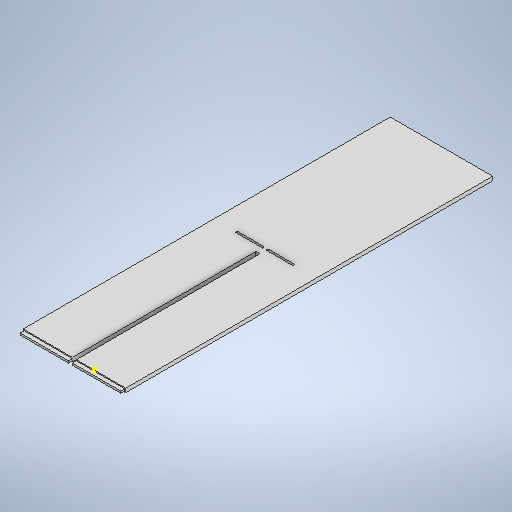
# Autodesk Inventor part: Sustainable Chair_V2 - Leg(A)_1_CPY
Saved by Autodesk Inventor 2025.2 (Build 292293000, 293)
## iProperties
Created: 2025-02-09
Part Number: Sustainable Chair_V2 - Leg(A)_1_CPY
Material: Foam Board - V3
Document SubType Name: Modeling
Designer: Dylan
Mass: 39.6007 g
Surface Area: 1188.97 cm^2
Volume: 262.027 cm^3
Density: 0.151132 g/cm^3
Appearance: Default(1)
Author: VRK99-0110
Title: Sustainable Chair_V2 - Leg(A)_1_CPY
Subject: Sustainable Chair Project
Autodesk Inventor part; units mm, degrees
ref_plane "YZ Plane" through (0, 0, 0) normal (1, 0, 0) x (0, 1, 0)
ref_plane "XZ Plane" through (0, 0, 0) normal (0, 1, 0) x (-1, 0, 0)
ref_plane "XY Plane" through (0, 0, 0) normal (0, 0, 1) x (1, 0, 0)
sketch "Sketch1" plane through (0, 0, 0) normal (0, 1, 0) x (-1, 0, 0)
  line L0 (0, 0) -> (50, 0)
  line L1 (50, 0) -> (50, -447.675)
  line L2 (50, -447.675) -> (0, -447.675)
  line L3 (0, -447.675) -> (0, 0)
  dimension "d0" = 50
  dimension "d1" = 447.675
  constraints: 8 end point, 2 parallel, 1 horizontal, 1 perpendicular
  measures "d0" distance of L1.end L2.end
  measures "d1" distance of L0.end L1.end
extrude "Extrusion1" add sketch "Sketch1" along normal blind 4.7625
sketch "Sketch2" plane through (-50, 0, 0) normal (0, 0, 1) x (1, 0, 0)
  line L0 (1.1907, 3.5648) -> (1.1907, 1.1907)
  line L1 (50, 0) -> (0, 0) projected
  line L2 (50, 4.7625) -> (0, 4.7625) projected
  line L3 (1.1907, 1.1907) -> (48.8093, 1.1907)
  line L4 (1.1907, 3.5648) -> (48.8093, 3.5648)
  line L5 (48.8093, 3.5648) -> (48.8093, 1.1907)
  line L6 (50, 0) -> (50, 4.7625) projected
  constraints: 8 end point, 1 parallel
extrude "Extrusion2" add sketch "Sketch2" along normal blind 4.7625
sketch "Sketch3" plane through (0, 4.7625, 0) normal (0, 1, 0) x (1, 0, 0)
  line L0 (-50, 447.675) -> (-50, 0) projected
  line L1 (-50, 447.675) -> (-25, 447.675)
  line L2 (0, 447.675) -> (-50, 447.675) projected
  line L3 (-25, 447.675) -> (-25, 382.675)
  line L4 (-31, 382.675) -> (-19, 382.675)
  line L5 (-31, 382.675) -> (-31, 0)
  line L6 (-1.1907, 0) -> (-48.8093, 0) projected
  line L7 (-19, 382.675) -> (-19, 0)
  line L8 (-31, 0) -> (-19, 0)
  point P0 (0, 0)
  dimension "d11" = 25
  constraints: 12 end point, 2 point on line, 2 vertical, 1 horizontal, 1 midpoint, 1 parallel, 1 perpendicular
  measures "d11" distance of L0.start L1.end
extrude "Extrusion3" cut sketch "Sketch3" against normal blind 10
sketch "Sketch4" plane through (-50, 0, 4.7625) normal (0, 0, 1) x (1, 0, 0)
  line L0 (31, 3.5648) -> (31, 1.1907) projected
  line L1 (31, 1.1907) -> (31, 3.5648)
  line L2 (19, 3.5648) -> (31, 3.5648) projected
  line L3 (31, 3.5648) -> (19, 3.5648)
  line L4 (19, 3.5648) -> (19, 1.1907)
  line L5 (19, 1.1907) -> (31, 1.1907)
  point P0 (50, 0)
  constraints: 8 end point, 3 perpendicular, 1 collinear
extrude "Extrusion4" cut sketch "Sketch4" against normal blind 10
sketch "Sketch5" plane through (0, 4.7625, 0) normal (0, 1, 0) x (1, 0, 0)
  point P0 (0, 0)
sketch "Sketch6" plane through (-31, 4.7625, -382.675) normal (0, 0, 1) x (1, 0, 0)
  line L0 (12, -4.7625) -> (0, -4.7625) projected
  line L1 (12, 0) -> (12, -4.7625) projected
  line L2 (0, 0) -> (12, 0) projected
  line L3 (0, 0) -> (0, -4.7625) projected
  point P0 (31, -4.7625)
extrude "Extrusion5" add sketch "Sketch6" along normal blind 158.838
sketch "Sketch8" plane through (-31, 4.7625, -223.837) normal (0, 0, 1) x (1, 0, 0)
  line L0 (3.6185, -4.7625) -> (3.6185, 0)
  line L1 (3.6185, 0) -> (8.3815, 0)
  line L2 (8.3815, 0) -> (8.3815, -4.7625)
  line L3 (3.6185, -4.7625) -> (8.3815, -4.7625)
  line L4 (0, -4.7625) -> (12, -4.7625) projected
  line L5 (-19, 0) -> (0, 0) projected
  line L6 (0, 0) -> (3.6185, 0)
  line L7 (12, 0) -> (0, 0) projected
  line L8 (3.6185, -4.7625) -> (0, -4.7625)
  line L9 (0, -4.7625) -> (0, 0) projected
  line L10 (0, -4.7625) -> (0, 0)
  line L11 (8.3815, 0) -> (12, 0)
  line L12 (12, -3.5718) -> (12, -4.7625) projected
  line L13 (12, -4.7625) -> (8.3815, -4.7625)
  line L14 (12, -4.7625) -> (12, 0)
  point P0 (31, -4.7625)
  dimension "d25" = 4.763
  constraints: 20 end point, 5 collinear, 3 perpendicular, 1 parallel
  measures "d25" distance of L0.end L1.end
extrude "Extrusion6" add sketch "Sketch8" along normal blind 223.837 contours L4 L9 L6 L0 | L2 L7 L14 L12 L4
sketch "Sketch9" plane through (-19, 1.1907, 0) normal (-1, 0, 0) x (0, 0, 1)
  line L0 (0, 2.374) -> (0, 0) projected
  line L1 (4.7625, 0) -> (0, 0) projected
  line L2 (4.7625, 2.374) -> (4.7625, 0) projected
  line L3 (0, 2.374) -> (4.7625, 2.374) projected
  point P0 (0, -1.1907)
extrude "Extrusion7" add sketch "Sketch9" along normal blind 15
sketch "Sketch10" plane through (-22.6185, 3.5648, 0) normal (0, 0, -1) x (-1, 0, 0)
  line L0 (4.763, -2.374) -> (4.763, 0) projected
  line L1 (0, 0) -> (4.763, 0) projected
  line L2 (0, 0) -> (0, -2.374) projected
  line L3 (0, -2.374) -> (4.763, -2.374) projected
  point P0 (-22.6185, -3.5648)
extrude "Extrusion8" cut sketch "Sketch10" against normal blind 15
sketch "Sketch14" plane through (0, 4.7625, 0) normal (0, 1, 0) x (1, 0, 0)
  line L0 (0, 447.675) -> (-50, 447.675) projected
  line L1 (0, 0) -> (0, 447.675) projected
  line L2 (-50, 447.675) -> (-50, 0) projected
  line L3 (-27.3815, 223.837) -> (-27.3815, 0) projected
  line L4 (-22.6185, 223.837) -> (-22.6185, 0) projected
  line L5 (-5, 231.488) -> (-22.6185, 231.488)
  line L6 (-22.6185, 231.488) -> (-22.6185, 233.862)
  line L7 (-22.6185, 233.862) -> (-5, 233.862)
  line L8 (-5, 231.488) -> (-5, 233.862)
  line L9 (-27.3815, 223.837) -> (-22.6185, 223.837) projected
  line L10 (-45, 231.488) -> (-27.3815, 231.488)
  line L11 (-27.3815, 231.488) -> (-27.3815, 233.862)
  line L12 (-27.3815, 233.862) -> (-45, 233.862)
  line L13 (-45, 231.488) -> (-45, 233.862)
  dimension "d35" = 2.374
  constraints: 16 end point, 1 perpendicular
  measures "d35" distance of L5.end L6.end
extrude "Extrusion9" cut sketch "Sketch14" against normal blind 10
sketch "Sketch17" plane through (0, 4.7625, 0) normal (0, 1, 0) x (1, 0, 0)
  line L0 (0, 0) -> (37.5, 0)
  line L1 (0, 447.675) -> (-50, 447.675) projected
  line L2 (0, 447.675) -> (37.5, 447.675)
  line L3 (37.5, 447.675) -> (37.5, 0)
  line L4 (0, 0) -> (0, 447.675) projected
  line L5 (0, 0) -> (0, 447.675)
  line L6 (-50, 0) -> (-87.5, 0)
  line L7 (-50, 447.675) -> (-87.5, 447.675)
  line L8 (-87.5, 447.675) -> (-87.5, 0)
  line L9 (-50, 0) -> (-50, 447.675)
  dimension "d39" = 37.5
  dimension "d40" = 37.5
  constraints: 16 end point, 2 horizontal, 1 collinear
  measures "d39" distance of L0.start L0.end
  measures "d40" distance of L1.start L2.end
extrude "Extrusion10" add sketch "Sketch17" against normal up to surface (4.7625 mm away)
sketch "Sketch18" plane through (-1.1907, 1.1907, 0) normal (0, 0, 1) x (1, 0, 0)
  line L0 (37.4997, 0) -> (0, 0)
  line L1 (0, 2.374) -> (0, 0) projected
  line L2 (0, 0) -> (0, 2.374)
  line L3 (0, 2.374) -> (37.4997, 2.374)
  line L4 (37.4997, 2.374) -> (37.4997, 0)
  line L5 (38.6907, -1.1907) -> (-86.3093, -1.1907) projected
  line L6 (-21.4278, 3.5718) -> (-26.1908, 3.5718) projected
  line L7 (-85.1183, 0) -> (-47.6185, 0)
  line L8 (-47.6185, 2.374) -> (-47.6185, 0)
  line L9 (-47.6185, 2.374) -> (-85.1183, 2.374)
  line L10 (-85.1183, 2.374) -> (-85.1183, 0)
  constraints: 16 end point, 2 perpendicular, 1 collinear
extrude "Extrusion11" add sketch "Sketch18" along normal up to surface (4.7625 mm away)
sketch "Sketch19" plane through (0, 4.7625, 0) normal (0, 1, 0) x (1, 0, 0)
  line L0 (-22.6185, 231.488) -> (9.8845, 231.488)
  line L1 (-22.6185, 233.862) -> (9.8845, 233.862)
  line L2 (9.8845, 233.862) -> (9.8845, 231.488)
  line L3 (-22.6185, 231.488) -> (-22.6185, 233.862)
  line L4 (-27.3815, 223.837) -> (-22.6185, 223.837) projected
  line L5 (-27.3815, 231.488) -> (-59.8845, 231.488)
  line L6 (-27.3815, 233.862) -> (-59.8845, 233.862)
  line L7 (-59.8845, 233.862) -> (-59.8845, 231.488)
  line L8 (-27.3815, 231.488) -> (-27.3815, 233.862)
  point P0 (0, 0)
  dimension "d47" = 32.503
  constraints: 16 end point, 1 horizontal
  measures "d47" distance of L1.start L1.end
extrude "Extrusion12" cut sketch "Sketch19" against normal blind 10
body "Solid1"
